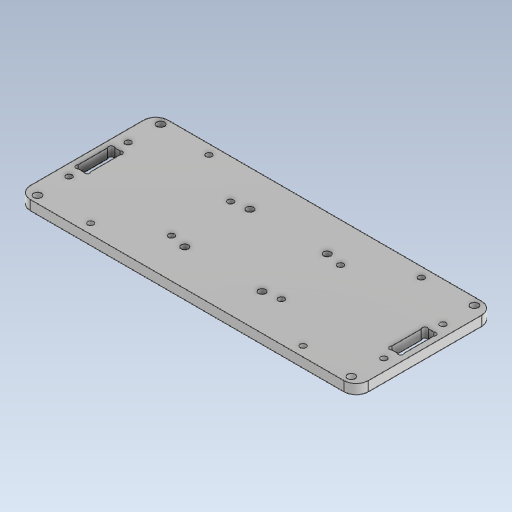
# Autodesk Inventor part: Trunk_lower_waisit_frame_
Saved by Autodesk Inventor 2020.4 (Build 244396000, 396)
## iProperties
Created: 2021-12-30
Part Number: Trunk_lower_waisit_frame_
Material: アルミニウム 2014-T4
Document SubType Name: Modeling
Designer: Masato Kubotera
Density: 2.8 g/cm^3
Appearance: 滑らか - 淡い灰色
Mass: 87.6968 g
Surface Area: 177.301 cm^2
Volume: 31.3203 cm^3
Author: Masato Kubotera
Autodesk Inventor part; units mm, degrees
ref_plane "YZ Plane" through (0, 0, 0) normal (1, 0, 0) x (0, 1, 0)
ref_plane "XZ Plane" through (0, 0, 0) normal (0, 1, 0) x (-1, 0, 0)
ref_plane "XY Plane" through (0, 0, 0) normal (0, 0, 1) x (1, 0, 0)
derived "Outer_support_stand.ipt"
sketch "スケッチ1" plane through (0, 0, 0) normal (0, 0, 1) x (1, 0, 0)
  circle A0 centre (0, 0) radius 18.5 construction
  circle A1 centre (0, 0) radius 20.5 construction
  circle A2 centre (0, 0) radius 20.51 construction
  line L0 (0, 0) -> (0, 24.5) construction
  circle A3 centre (0, 24.5) radius 1.55 construction
  circle A4 centre (0, 24.5) radius 3 construction
  arc A5 (0, 28.5) -> (-3.7147, 25.9835) centre (0, 24.5) ccw construction
  arc A6 (-5.1639, 24.7674) -> (-18.8673, 16.8557) centre (0, 0) ccw construction
  arc A7 (-5.1639, 24.7674) -> (-3.7147, 25.9835) centre (-5.5721, 26.7253) ccw construction
  arc A8 (3.7147, 25.9835) -> (5.1639, 24.7674) centre (5.5721, 26.7253) ccw construction
  arc A9 (3.7147, 25.9835) -> (0, 28.5) centre (0, 24.5) ccw construction
  circle A10 centre (0, 24.5) radius 3.05 construction
  arc A11 (-24.0311, 7.9117) -> (-24.0311, -7.9117) centre (0, 0) ccw construction
  arc A12 (-24.0311, 7.9117) -> (-24.3598, 9.7747) centre (-25.9308, 8.5371) ccw construction
  arc A13 (-24.6817, 14.25) -> (-24.3598, 9.7747) centre (-21.2176, 12.25) ccw construction
  arc A14 (-20.645, 16.2088) -> (-24.6817, 14.25) centre (-21.2176, 12.25) ccw construction
  arc A15 (-20.645, 16.2088) -> (-18.8673, 16.8557) centre (-20.3588, 18.1882) ccw construction
  circle A16 centre (-21.2176, 12.25) radius 3.05 construction
  circle A17 centre (-21.2176, 12.25) radius 1.55 construction
  arc A18 (-18.8673, -16.8557) -> (-5.1639, -24.7674) centre (0, 0) ccw construction
  arc A19 (-18.8673, -16.8557) -> (-20.645, -16.2088) centre (-20.3588, -18.1882) ccw construction
  arc A20 (-24.6817, -14.25) -> (-20.645, -16.2088) centre (-21.2176, -12.25) ccw construction
  arc A21 (-24.3598, -9.7747) -> (-24.6817, -14.25) centre (-21.2176, -12.25) ccw construction
  arc A22 (-24.3598, -9.7747) -> (-24.0311, -7.9117) centre (-25.9308, -8.5371) ccw construction
  circle A23 centre (-21.2176, -12.25) radius 3.05 construction
  circle A24 centre (-21.2176, -12.25) radius 1.55 construction
  arc A25 (5.1639, -24.7674) -> (18.8673, -16.8557) centre (0, 0) ccw construction
  arc A26 (5.1639, -24.7674) -> (3.7147, -25.9835) centre (5.5721, -26.7253) ccw construction
  arc A27 (0, -28.5) -> (3.7147, -25.9835) centre (0, -24.5) ccw construction
  arc A28 (-3.7147, -25.9835) -> (0, -28.5) centre (0, -24.5) ccw construction
  arc A29 (-3.7147, -25.9835) -> (-5.1639, -24.7674) centre (-5.5721, -26.7253) ccw construction
  circle A30 centre (0, -24.5) radius 3.05 construction
  circle A31 centre (0, -24.5) radius 1.55 construction
  arc A32 (24.0311, -7.9117) -> (24.0311, 7.9117) centre (0, 0) ccw construction
  arc A33 (24.0311, -7.9117) -> (24.3598, -9.7747) centre (25.9308, -8.5371) ccw construction
  arc A34 (24.6817, -14.25) -> (24.3598, -9.7747) centre (21.2176, -12.25) ccw construction
  arc A35 (20.645, -16.2088) -> (24.6817, -14.25) centre (21.2176, -12.25) ccw construction
  arc A36 (20.645, -16.2088) -> (18.8673, -16.8557) centre (20.3588, -18.1882) ccw construction
  circle A37 centre (21.2176, -12.25) radius 3.05 construction
  circle A38 centre (21.2176, -12.25) radius 1.55 construction
  arc A39 (18.8673, 16.8557) -> (5.1639, 24.7674) centre (0, 0) ccw construction
  arc A40 (18.8673, 16.8557) -> (20.645, 16.2088) centre (20.3588, 18.1882) ccw construction
  arc A41 (24.6817, 14.25) -> (20.645, 16.2088) centre (21.2176, 12.25) ccw construction
  arc A42 (24.3598, 9.7747) -> (24.6817, 14.25) centre (21.2176, 12.25) ccw construction
  arc A43 (24.3598, 9.7747) -> (24.0311, 7.9117) centre (25.9308, 8.5371) ccw construction
  circle A44 centre (21.2176, 12.25) radius 3.05 construction
  circle A45 centre (21.2176, 12.25) radius 1.55 construction
sketch "スケッチ2" plane through (0, 0, 0) normal (0, 0, 1) x (1, 0, 0)
  line L0 (-114, 28.5) -> (26, 28.5)
  line L1 (26, 28.5) -> (26, -28.5)
  line L2 (26, -28.5) -> (-114, -28.5)
  line L3 (-114, -28.5) -> (-114, 28.5)
  line L4 (-114, 28.5) -> (26, -28.5) construction
  line L5 (26, 28.5) -> (-114, -28.5) construction
  line L6 (-114, 0) -> (26, 0) construction
  line L7 (-44, 28.5) -> (-44, -28.5) construction
  line L8 (18.5, 7.5) -> (23.5, 7.5) construction
  line L9 (23.5, 7.5) -> (23.5, -7.5) construction
  line L10 (23.5, -7.5) -> (18.5, -7.5) construction
  line L11 (18.5, -7.5) -> (18.5, 7.5) construction
  line L12 (18.5, 7.5) -> (23.5, -7.5) construction
  line L13 (23.5, 7.5) -> (18.5, -7.5) construction
  circle A0 centre (21, -25.5) radius 1.6
  circle A1 centre (0, 0) radius 10.5 construction
  line L14 (-28, 13.5) -> (-1, 13.5) construction
  line L15 (-1, 13.5) -> (-1, -13.5) construction
  line L16 (-1, -13.5) -> (-28, -13.5) construction
  line L17 (-28, -13.5) -> (-28, 13.5) construction
  line L18 (-28, 13.5) -> (-1, -13.5) construction
  line L19 (-1, 13.5) -> (-28, -13.5) construction
  line L20 (13, 16) -> (-38.5, 16) construction
  line L21 (-38.5, 16) -> (-38.5, -16) construction
  line L22 (-38.5, -16) -> (13, -16) construction
  line L23 (13, -16) -> (13, 16) construction
  line L24 (13, 16) -> (-38.5, -16) construction
  line L25 (-38.5, 16) -> (13, -16) construction
  circle A2 centre (-28, -13.5) radius 2.5 construction
  line L26 (18.45, 7.55) -> (23.55, 7.55)
  line L27 (23.55, 7.55) -> (23.55, -7.55)
  line L28 (23.55, -7.55) -> (18.45, -7.55)
  line L29 (18.45, -7.55) -> (18.45, 7.55)
  line L30 (18.45, 7.55) -> (23.55, -7.55) construction
  line L31 (23.55, 7.55) -> (18.45, -7.55) construction
  arc A3 (19.9349, 7.55) -> (18.45, 6.0651) centre (19.1925, 6.8075) ccw
  line L32 (21, 7.5) -> (21, -7.5) construction
  line L33 (18.5, 0) -> (23.5, 0) construction
  arc A4 (23.55, 6.0651) -> (22.0651, 7.55) centre (22.8075, 6.8075) ccw
  arc A5 (18.45, -6.0651) -> (19.9349, -7.55) centre (19.1925, -6.8075) ccw
  arc A6 (22.0651, -7.55) -> (23.55, -6.0651) centre (22.8075, -6.8075) ccw
  circle A7 centre (-28, -13.5) radius 1.5
  circle A8 centre (-28, 13.5) radius 1.5
  circle A9 centre (0, 24.5) radius 1.55 construction
  circle A10 centre (-21.2176, 12.25) radius 1.55 construction
  circle A11 centre (-21.2176, -12.25) radius 1.55 construction
  circle A12 centre (0, -24.5) radius 1.55 construction
  circle A13 centre (21.2176, -12.25) radius 1.55 construction
  circle A14 centre (21.2176, 12.25) radius 1.55 construction
  circle A15 centre (0, 24.5) radius 1.25
  circle A16 centre (-21.2176, 12.25) radius 1.25
  circle A17 centre (-21.2176, -12.25) radius 1.25
  circle A18 centre (0, -24.5) radius 1.25
  circle A19 centre (21.2176, -12.25) radius 1.25
  circle A20 centre (21.2176, 12.25) radius 1.25
  arc A21 (21, -28.5) -> (26, -23.5) centre (21, -23.5) ccw
  circle A22 centre (21, 25.5) radius 1.6
  arc A23 (26, 23.5) -> (21, 28.5) centre (21, 23.5) ccw
  circle A24 centre (-109, -25.5) radius 1.6
  line L34 (-106.45, 7.55) -> (-111.55, 7.55)
  line L35 (-111.55, 7.55) -> (-111.55, -7.55)
  line L36 (-111.55, -7.55) -> (-106.45, -7.55)
  line L37 (-106.45, -7.55) -> (-106.45, 7.55)
  arc A25 (-106.45, 6.0651) -> (-107.9349, 7.55) centre (-107.1925, 6.8075) ccw
  arc A26 (-110.0651, 7.55) -> (-111.55, 6.0651) centre (-110.8075, 6.8075) ccw
  arc A27 (-107.9349, -7.55) -> (-106.45, -6.0651) centre (-107.1925, -6.8075) ccw
  arc A28 (-111.55, -6.0651) -> (-110.0651, -7.55) centre (-110.8075, -6.8075) ccw
  circle A29 centre (-60, -13.5) radius 1.5
  circle A30 centre (-60, 13.5) radius 1.5
  circle A31 centre (-88, 24.5) radius 1.25
  circle A32 centre (-66.7824, 12.25) radius 1.25
  circle A33 centre (-66.7824, -12.25) radius 1.25
  circle A34 centre (-88, -24.5) radius 1.25
  circle A35 centre (-109.2176, -12.25) radius 1.25
  circle A36 centre (-109.2176, 12.25) radius 1.25
  arc A37 (-114, -23.5) -> (-109, -28.5) centre (-109, -23.5) ccw
  circle A38 centre (-109, 25.5) radius 1.6
  arc A39 (-109, 28.5) -> (-114, 23.5) centre (-109, 23.5) ccw
  point P0 (-44, 0)
  point P1 (0, 28.5)
  point P2 (0, -28.5)
  point P3 (21, 0)
  point P4 (-14.5, 0)
  point P5 (-12.75, 0)
  point P6 (21, 0)
  point P7 (22.0651, -7.55)
  point P8 (19.9349, -7.55)
  point P9 (18.45, -6.0651)
  point P10 (22.0651, 7.55)
  point P11 (23.55, -6.0651)
  point P12 (-110.0651, 7.55)
  point P13 (-106.45, -6.0651)
  point P14 (-107.9349, -7.55)
  point P15 (-110.0651, -7.55)
  point P16 (-111.55, -6.0651)
  point P17 (-111.55, 6.0651)
  dimension "d1" = 57
  dimension "d2" = 57
  dimension "d4" = 44
  dimension "d5" = 5
  dimension "d6" = 15
  dimension "d7" = 3.2
  dimension "d8" = 21
  dimension "d9" = 27
  dimension "d10" = 27
  dimension "d11" = 1
  dimension "d13" = 5
  dimension "d14" = 0.05
  dimension "d15" = 0.05
  dimension "d16" = 1.05
  dimension "d17" = 3
  dimension "d19" = 62.5
  dimension "d20" = 2.5
  dimension "d21" = 3
  dimension "d22" = 32
  dimension "d23" = 51.5
  dimension "d24" = 13
  dimension "d25" = 2.5
  dimension "d26" = 2.5
  dimension "d27" = 2.5
  dimension "d28" = 2.5
  dimension "d29" = 2.5
  dimension "d30" = 2.5
  constraints: 76 end point, 46 symmetric about line, 34 centre point, 25 point on circle, 19 midpoint, 12 point on line, 10 parallel, 9 coincident, 5 horizontal, 5 perpendicular, 2 tangent, 22 other
  measures "d1" distance of point (0, -28.5) point (0, 28.5)
  measures "d2" distance of L0.end L1.end
  measures "d4" distance of point (-44, 0) point (0, 0)
  measures "d5" distance of L9.end L10.end
  measures "d6" distance of L8.end L9.end
  measures "d7" diameter of A0
  measures "d8" diameter of A1
  measures "d9" distance of L15.end L16.end
  measures "d10" distance of L14.end L15.end
  measures "d11" distance from line of L15 point (0, 0)
  measures "d13" diameter of A2
  measures "d14" distance between parallel lines of L29 L11
  measures "d15" distance between parallel lines of L26 L8
  measures "d16" radius of A3
  measures "d17" distance from line of L2 A0.centre
  measures "d19" distance between parallel lines of L11 L7
  measures "d20" distance of L6.end L33.end
  measures "d21" diameter of A7
  measures "d22" distance of L22.end L20.start
  measures "d23" distance of L20.start L20.end
  measures "d24" distance from line of L23 point (0, 0)
  measures "d25" diameter of A15
  measures "d26" diameter of A16
  measures "d27" diameter of A17
  measures "d28" diameter of A18
  measures "d29" diameter of A19
  measures "d30" diameter of A20
extrude "押し出し1" add sketch "スケッチ2" along normal blind 4 contours L0 A23 L1 A21 L2 A37 L3 A39
equation "\"d2\" = d1"
equation "\"d15\" = d14"
